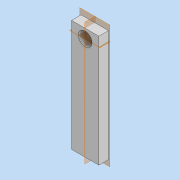
# Autodesk Inventor part: bearing1
Saved by Autodesk Inventor 2022 (Build 260153000, 153)
## iProperties
Created: 2023-12-21
Part Number: bearing1
Material: 一般
Document SubType Name: Modeling
Designer: ktamu
Density: 1 g/cm^3
Appearance: 既定
Author: ktamu
Autodesk Inventor part; units mm, degrees
sketch "スケッチ1" plane through (0, 0, 0) normal (0, 0, 1) x (1, 0, 0)
  circle A0 centre (0, 0) radius 10
  line L0 (20, -150) -> (20, 13.4743)
  line L1 (20, 13.4743) -> (-20, 13.4743)
  line L2 (-20, 13.4743) -> (-20, -150)
  line L3 (-20, -150) -> (20, -150)
  line L4 (20, -150) -> (-20, 13.4743) construction
  line L5 (20, 13.4743) -> (-20, -150) construction
  line L6 (-28, 0) -> (28, 0) projected
  point P0 (0, -68.2629)
  dimension "d0" = 20
  dimension "d1" = 40
  dimension "d4" = 150
  constraints: 12 end point, 2 midpoint, 2 parallel, 1 centre point, 1 coincident, 1 perpendicular, 1 vertical
  measures "d0" diameter of A0
  measures "d1" distance of L1.end L0.end
  measures "d4" distance between parallel lines of L3 L6
extrude "押し出し1" add sketch "スケッチ1" along normal blind 14 contours L6 L0 L3 L2 A0 | A0 L6 L2 L1 L0
sketch "スケッチ2" plane through (-20, -150, 0) normal (0, -1, 0) x (1, 0, 0)
  point P0 (20, 0)
